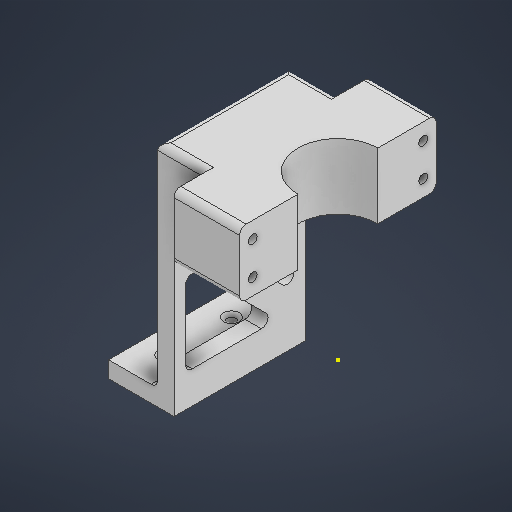
# Autodesk Inventor part: alt blok
Saved by Autodesk Inventor 2026.1 (Build 301233020, 233B)
## iProperties
Created: 2026-04-16
Part Number: alt blok
Material: Generic
Document SubType Name: Modeling
Designer: kadir
Density: 1 g/cm^3
Appearance: Default
Author: kadir
Autodesk Inventor part; units mm, degrees
ref_plane "YZ Plane" through (0, 0, 0) normal (1, 0, 0) x (0, 1, 0)
ref_plane "XZ Plane" through (0, 0, 0) normal (0, 1, 0) x (-1, 0, 0)
ref_plane "XY Plane" through (0, 0, 0) normal (0, 0, 1) x (1, 0, 0)
sketch "Sketch1" plane through (0, 0, 0) normal (0, 0, 1) x (1, 0, 0)
  line L0 (0, 0) -> (20, 0)
  line L1 (20, 0) -> (20, 5)
  line L2 (14.9919, 5) -> (0, 5)
  line L3 (0, 5) -> (0, 0)
  line L4 (20, 0) -> (10.3687, 0)
  line L5 (14.9919, 5) -> (14.9919, 69.8472)
  line L6 (14.9919, 69.8472) -> (24.9919, 69.8472)
  line L7 (20, 49.8472) -> (20, 0)
  line L8 (14.9919, 69.8472) -> (49.9915, 69.8472)
  line L9 (49.9915, 69.8472) -> (49.9915, 49.8472)
  line L10 (49.9915, 49.8472) -> (20, 49.8472)
  line L11 (14.9919, 50) -> (14.9919, 69.8472)
  dimension "d0" = 20
  dimension "d1" = 5
  dimension "d2" = 10
  dimension "d4" = 35
  dimension "d5" = 20
  dimension "d37" = 64.8472
  dimension "d38" = 49.8472
  constraints: 24 end point, 6 parallel, 3 horizontal, 3 perpendicular
  measures "d0" distance of L2.end L1.end
  measures "d1" distance of L1.end L0.end
  measures "d2" distance of L5.end L6.end
  measures "d4" distance of L9.end L11.start
  measures "d5" distance of L8.end L9.end
  measures "d37" distance of L2.start L5.end
  measures "d38" distance of L7.start L0.end
extrude "Extrusion1" add sketch "Sketch1" along normal blind 40
sketch "Sketch2" plane through (14.9919, 69.8472, 0) normal (0, 1, 0) x (1, 0, 0)
  line L0 (34.9997, 0) -> (34.9997, -40) projected
  circle A0 centre (34.9997, -20) radius 12.2
  point P0 (-14.9919, 0)
  point P1 (34.9997, -32.2)
  point P2 (34.9997, -7.8)
  dimension "d8" = 24.4
  constraints: 1 centre point, 1 midpoint
  measures "d8" diameter of A0
extrude "Extrusion2" cut sketch "Sketch2" against normal blind 30 contours L0 A0 picked at (30.3566, -23.0439)
sketch "Sketch4" plane through (0, 0, 40) normal (0, 0, 1) x (1, 0, 0)
  line L0 (49.9915, 69.8472) -> (14.9919, 69.8472) projected
  line L1 (49.9915, 69.8472) -> (29.9915, 69.8472)
  line L2 (29.9915, 69.8472) -> (29.9915, 49.8472)
  line L3 (29.9915, 49.8472) -> (49.9915, 49.8472)
  line L4 (49.9915, 49.8472) -> (49.9915, 69.8472)
  point P0 (0, 0)
  dimension "d17" = 20
  dimension "d18" = 20
  constraints: 8 end point, 2 parallel, 1 horizontal, 1 perpendicular
  measures "d17" distance of L3.end L2.end
  measures "d18" distance of L2.end L1.end
extrude "Extrusion4" add sketch "Sketch4" along normal blind 10
sketch "Sketch5" plane through (0, 0, 0) normal (0, 0, -1) x (-1, 0, 0)
  line L0 (-49.9915, 49.8472) -> (-49.9915, 69.8472) projected
  line L1 (-49.9915, 69.8472) -> (-29.9915, 69.8472)
  line L2 (-29.9915, 69.8472) -> (-29.9915, 49.8472)
  line L3 (-29.9915, 49.8472) -> (-49.9915, 49.8472)
  line L4 (-49.9915, 49.8472) -> (-49.9915, 69.8472)
  point P0 (0, 0)
  dimension "d21" = 20
  dimension "d22" = 20
  constraints: 8 end point, 2 parallel, 1 horizontal, 1 perpendicular
  measures "d21" distance of L2.end L3.end
  measures "d22" distance of L1.end L2.end
extrude "Extrusion5" add sketch "Sketch5" along normal blind 10
sketch "Sketch6" plane through (49.9915, 49.8472, 32.2) normal (1, 0, 0) x (0, 0, -1)
  circle A0 centre (-13.8, 15) radius 1.35
  line L0 (-17.8, 0) -> (-17.8, 20) projected
  line L1 (0, 20) -> (-17.8, 20) projected
  line L2 (-17.8, 10) -> (42.2, 10)
  line L3 (42.2, 0) -> (42.2, 20) projected
  circle A1 centre (-13.8, 5) radius 1.35
  line L4 (32.2, 20) -> (-7.8, 20) projected
  line L5 (12.2, 20) -> (12.2, 0)
  line L6 (32.2, 0) -> (-7.8, 0) projected
  circle A2 centre (38.2, 15) radius 1.35
  circle A3 centre (38.2, 5) radius 1.35
  point P0 (32.2, -49.8472)
  dimension "d25" = 2.7
  dimension "d26" = 4
  dimension "d27" = 5
  constraints: 4 centre point, 4 end point, 4 midpoint, 3 symmetric about line, 3 other
  measures "d25" diameter of A0
  measures "d26" distance from line of L0 A0.centre
  measures "d27" distance from line of L1 A0.centre
extrude "Extrusion6" cut sketch "Sketch6" against normal through all contours A0 | A1 | A2 | A3
sketch "Sketch7" plane through (0, 5, 0) normal (0, 1, 0) x (1, 0, 0)
  circle A0 centre (7.5, -30) radius 1.4
  line L0 (0, 0) -> (0, -40) projected
  line L1 (14.9919, -40) -> (0, -40) projected
  line L2 (14.9919, 0) -> (14.9919, -40) projected
  line L3 (14.9919, -20) -> (0, -20)
  circle A1 centre (7.5, -10) radius 1.4
  dimension "d30" = 2.8
  dimension "d31" = 7.5
  dimension "d32" = 10
  constraints: 2 centre point, 2 end point, 2 midpoint, 1 symmetric about line, 1 other
  measures "d30" diameter of A0
  measures "d31" distance from line of L0 A0.centre
  measures "d32" distance from line of L1 A0.centre
extrude "Extrusion7" cut sketch "Sketch7" against normal through all contours A0 | A1
fillet "Fillet1" radius 2 2 edges at (39.9915, 69.8472, 50) (39.9915, 49.8472, 50)
fillet "Fillet2" radius 2 1 edges at (39.9915, 69.8472, -10)
fillet "Fillet3" radius 2 1 edges at (39.9915, 49.8472, -10)
fillet "Fillet4" radius 2 3 edges at (22.4917, 69.8472, 40) (22.4917, 69.8472, 0) (14.9919, 69.8472, 20)
fillet "Fillet5" radius 1 1 edges at (6.1, 5, 10)
fillet "Fillet6" radius 1 1 edges at (6.1, 5, 30)
fillet "Fillet7" radius 1 2 edges at (29.9915, 64.8472, -4.65) (29.9915, 54.8472, -4.65)
fillet "Fillet8" radius 1 2 edges at (29.9915, 64.8472, 47.35) (29.9915, 54.8472, 47.35)
sketch "Sketch8" plane through (14.9919, 5, 0) normal (-1, 0, 0) x (0, 0, 1)
  line L0 (0, -5) -> (0, 44.8472) projected
  line L1 (0, 0) -> (40, 0) projected
  line L2 (0, 44.8472) -> (40, 44.8472)
  line L3 (40, 44.8472) -> (40, 0)
  line L4 (40, 0) -> (0, 0)
  line L5 (0, 0) -> (0, 44.8472)
  line L6 (3.5, 37.8472) -> (36.5, 37.8472)
  line L7 (36.5, 37.8472) -> (36.5, 4.8472)
  line L8 (36.5, 4.8472) -> (3.5, 4.8472)
  line L9 (3.5, 4.8472) -> (3.5, 37.8472)
  line L10 (31.5, 37.8472) -> (3.5, 9.8472)
  line L11 (36.5, 32.8472) -> (8.5, 4.8472)
  point P0 (36.5, 21.3472)
  dimension "d47" = 33
  dimension "d48" = 33
  dimension "d49" = 3.5
  dimension "d50" = 7
  dimension "d51" = 5
  dimension "d52" = 5
  dimension "d53" = 5
  dimension "d54" = 5
  constraints: 20 end point, 4 parallel, 4 point on line, 2 horizontal, 2 perpendicular, 1 midpoint
  measures "d47" distance of L7.end L8.end
  measures "d48" distance of L6.end L7.end
  measures "d49" distance from line of L3 point (36.5, 21.347)
  measures "d50" distance between parallel lines of L2 L6
  measures "d51" distance of L6.end L10.start
  measures "d52" distance of L8.end L10.end
  measures "d53" distance of L6.end L11.start
  measures "d54" distance of L8.end L11.end
extrude "Extrusion8" cut sketch "Sketch8" against normal blind 10 contours L6 L10 L9 | L7 L8 L11
fillet "Fillet9" radius 2 2 edges at (17.4959, 9.8472, 36.5) (17.4959, 9.8472, 8.5)
fillet "Fillet10" radius 2 1 edges at (17.4959, 14.8472, 3.5)
fillet "Fillet11" radius 2 1 edges at (17.4959, 42.8472, 31.5)
fillet "Fillet12" radius 2 1 edges at (17.4959, 42.8472, 3.5)
fillet "Fillet13" radius 2 1 edges at (17.4959, 37.8472, 36.5)
fillet "Fillet14" radius 2 1 edges at (14.9919, 5, 20)
sketch "Sketch9" plane through (29.9915, 51.8472, -10) normal (-1, 0, 0) x (0, 0, 1)
  point P0 (10, -51.8472)
sketch "Sketch10" plane through (29.9915, 51.8472, -10) normal (-1, 0, 0) x (0, 0, 1)
  point P0 (10, -51.8472)
sketch "Sketch11" plane through (29.9915, 51.8472, 50) normal (-1, 0, 0) x (0, 0, 1)
  point P0 (-50, -51.8472)
sketch "Sketch12" plane through (0, 5, 40) normal (0, 1, 0) x (1, 0, 0)
  point P0 (0, 40)
body "Solid1"
